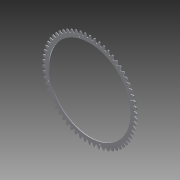
# Autodesk Inventor part: Large Spur Gear
Saved by Autodesk Inventor 2014 SP1 (Build 180222100, 222)
## iProperties
Created: 2012-03-30
Part Number: Large Spur Gear
Material: Aluminum-6061
Document SubType Name: Modeling
Designer: Moses
Mass: 183.263 g
Surface Area: 529.591 cm^2
Volume: 67.6246 cm^3
Density: 2.71 g/cm^3
Appearance: Aluminum - Flat
Author: Moses
Autodesk Inventor part; units mm, degrees
ref_plane "YZ Plane" through (0, 0, 0) normal (1, 0, 0) x (0, 1, 0)
ref_plane "XZ Plane" through (0, 0, 0) normal (0, 1, 0) x (-1, 0, 0)
ref_plane "XY Plane" through (0, 0, 0) normal (0, 0, 1) x (1, 0, 0)
sketch "Sketch1" plane through (0, 0, 0) normal (0, 0, 1) x (1, 0, 0)
  arc A0 (-21.3828, 186.7398) -> (-24.453, 174.3486) centre (39.2428, 165.1423) ccw
  arc A1 (-24.453, 174.3486) -> (-28.8619, 173.6732) centre (0, 0) ccw
  arc A2 (-28.8619, 173.6732) -> (-35.5008, 184.577) centre (-86.8806, 145.8209) ccw
  arc A3 (-35.5008, 184.577) -> (-40.1653, 183.6184) centre (0, 0) ccw
  arc A4 (-40.1653, 183.6184) -> (-41.9661, 170.9802) centre (22.3343, 168.2651) ccw
  arc A5 (-41.9661, 170.9802) -> (-46.2841, 169.8622) centre (0, 0) ccw
  arc A6 (-46.2841, 169.8622) -> (-53.992, 180.0384) centre (-101.1873, 136.2831) ccw
  arc A7 (-53.992, 180.0384) -> (-58.5355, 178.6129) centre (0, 0) ccw
  arc A8 (-58.5355, 178.6129) -> (-59.0486, 165.8573) centre (5.1966, 169.6613) ccw
  arc A9 (-59.0486, 165.8573) -> (-63.2313, 164.3082) centre (0, 0) ccw
  arc A10 (-63.2313, 164.3082) -> (-71.9292, 173.6524) centre (-114.4557, 125.347) ccw
  arc A11 (-71.9292, 173.6524) -> (-76.3052, 171.7745) centre (0, 0) ccw
  arc A12 (-76.3052, 171.7745) -> (-75.5251, 159.0325) centre (-11.9944, 169.3166) ccw
  arc A13 (-75.5251, 159.0325) -> (-79.5296, 157.0682) centre (0, 0) ccw
  arc A14 (-79.5296, 157.0682) -> (-89.1283, 165.4845) centre (-126.5496, 113.1245) ccw
  arc A15 (-89.1283, 165.4845) -> (-93.2918, 163.1735) centre (0, 0) ccw
  arc A16 (-93.2918, 163.1735) -> (-91.2267, 150.5758) centre (-29.0623, 167.2344) ccw
  arc A17 (-91.2267, 150.5758) -> (-95.0119, 148.2164) centre (0, 0) ccw
  arc A18 (-95.0119, 148.2164) -> (-105.4128, 155.6185) centre (-137.3449, 99.7413) ccw
  arc A19 (-105.4128, 155.6185) -> (-109.3212, 152.8982) centre (0, 0) ccw
  arc A20 (-109.3212, 152.8982) -> (-105.9921, 140.574) centre (-45.832, 163.4362) ccw
  arc A21 (-105.9921, 140.574) -> (-109.5192, 137.8438) centre (0, 0) ccw
  arc A22 (-109.5192, 137.8438) -> (-120.6156, 144.1556) centre (-146.7309, 85.3346) ccw
  arc A23 (-120.6156, 144.1556) -> (-124.2287, 141.0538) centre (0, 0) ccw
  arc A24 (-124.2287, 141.0538) -> (-119.67, 129.1297) centre (-62.1314, 157.9609) ccw
  arc A25 (-119.67, 129.1297) -> (-122.9028, 126.0567) centre (0, 0) ccw
  arc A26 (-122.9028, 126.0567) -> (-134.5807, 131.2135) centre (-154.6113, 70.0523) ccw
  arc A27 (-134.5807, 131.2135) -> (-137.8615, 127.7621) centre (0, 0) ccw
  arc A28 (-137.8615, 127.7621) -> (-132.1198, 116.3604) centre (-77.7933, 150.8647) ccw
  arc A29 (-132.1198, 116.3604) -> (-135.0251, 112.9761) centre (0, 0) ccw
  arc A30 (-135.0251, 112.9761) -> (-147.1649, 116.925) centre (-160.9051, 54.0511) ccw
  arc A31 (-147.1649, 116.925) -> (-150.0797, 113.1594) centre (0, 0) ccw
  arc A32 (-150.0797, 113.1594) -> (-143.2139, 102.397) centre (-92.6569, 142.2205) ccw
  arc A33 (-143.2139, 102.397) -> (-145.762, 98.7361) centre (0, 0) ccw
  arc A34 (-145.762, 98.7361) -> (-158.2389, 101.4367) centre (-165.5478, 37.4953) ccw
  arc A35 (-158.2389, 101.4367) -> (-160.7578, 97.3955) centre (0, 0) ccw
  arc A36 (-160.7578, 97.3955) -> (-152.8385, 87.3829) centre (-106.5697, 132.1168) ccw
  arc A37 (-152.8385, 87.3829) -> (-155.0031, 83.4831) centre (0, 0) ccw
  arc A38 (-155.0031, 83.4831) -> (-167.6892, 84.9075) centre (-168.4917, 20.5547) ccw
  arc A39 (-167.6892, 84.9075) -> (-169.7864, 80.6322) centre (0, 0) ccw
  arc A40 (-169.7864, 80.6322) -> (-160.8947, 71.4722) centre (-119.389, 120.6575) ccw
  arc A41 (-160.8947, 71.4722) -> (-162.6536, 67.3733) centre (0, 0) ccw
  arc A42 (-162.6536, 67.3733) -> (-175.4188, 67.507) centre (-169.7068, 3.4032) ccw
  arc A43 (-175.4188, 67.507) -> (-177.0727, 63.0415) centre (0, 0) ccw
  arc A44 (-177.0727, 63.0415) -> (-167.2999, 54.828) centre (-130.9832, 107.9601) ccw
  arc A45 (-167.2999, 54.828) -> (-168.6352, 50.5723) centre (0, 0) ccw
  arc A46 (-168.6352, 50.5723) -> (-181.3484, 49.4138) centre (-169.1803, -13.7832) ccw
  arc A47 (-181.3484, 49.4138) -> (-182.542, 44.8039) centre (0, 0) ccw
  arc A48 (-182.542, 44.8039) -> (-171.9884, 37.6213) centre (-141.2333, 94.1548) ccw
  arc A49 (-171.9884, 37.6213) -> (-172.8863, 33.2523) centre (0, 0) ccw
  arc A50 (-172.8863, 33.2523) -> (-185.4171, 30.8136) centre (-166.9179, -30.8281) ccw
  arc A51 (-185.4171, 30.8136) -> (-186.1381, 26.1066) centre (0, 0) ccw
  arc A52 (-186.1381, 26.1066) -> (-174.9121, 20.0285) centre (-150.0341, 79.3834) ccw
  arc A53 (-174.9121, 20.0285) -> (-175.3633, 15.5911) centre (0, 0) ccw
  arc A54 (-175.3633, 15.5911) -> (-187.5831, 11.8972) centre (-162.9427, -47.5568) ccw
  arc A55 (-187.5831, 11.8972) -> (-187.8243, 7.1414) centre (0, 0) ccw
  arc A56 (-187.8243, 7.1414) -> (-176.0409, 2.2302) centre (-157.2954, 63.7974) ccw
  arc A57 (-176.0409, 2.2302) -> (-176.0409, -2.2302) centre (0, 0) ccw
  arc A58 (-176.0409, -2.2302) -> (-187.8243, -7.1414) centre (-157.2954, -63.7974) ccw
  arc A59 (-187.8243, -7.1414) -> (-187.5831, -11.8972) centre (0, 0) ccw
  arc A60 (-187.5831, -11.8972) -> (-175.3633, -15.5911) centre (-162.9427, 47.5568) ccw
  arc A61 (-175.3633, -15.5911) -> (-174.9121, -20.0285) centre (0, 0) ccw
  arc A62 (-174.9121, -20.0285) -> (-186.1381, -26.1066) centre (-150.0341, -79.3834) ccw
  arc A63 (-186.1381, -26.1066) -> (-185.4171, -30.8136) centre (0, 0) ccw
  arc A64 (-185.4171, -30.8136) -> (-172.8863, -33.2523) centre (-166.9179, 30.8281) ccw
  arc A65 (-172.8863, -33.2523) -> (-171.9884, -37.6213) centre (0, 0) ccw
  arc A66 (-171.9884, -37.6213) -> (-182.542, -44.8039) centre (-141.2333, -94.1548) ccw
  arc A67 (-182.542, -44.8039) -> (-181.3484, -49.4138) centre (0, 0) ccw
  arc A68 (-181.3484, -49.4138) -> (-168.6352, -50.5723) centre (-169.1803, 13.7832) ccw
  arc A69 (-168.6352, -50.5723) -> (-167.2999, -54.828) centre (0, 0) ccw
  arc A70 (-167.2999, -54.828) -> (-177.0727, -63.0415) centre (-130.9832, -107.9601) ccw
  arc A71 (-177.0727, -63.0415) -> (-175.4188, -67.507) centre (0, 0) ccw
  arc A72 (-175.4188, -67.507) -> (-162.6536, -67.3733) centre (-169.7068, -3.4032) ccw
  arc A73 (-162.6536, -67.3733) -> (-160.8947, -71.4722) centre (0, 0) ccw
  arc A74 (-160.8947, -71.4722) -> (-169.7864, -80.6322) centre (-119.389, -120.6575) ccw
  arc A75 (-169.7864, -80.6322) -> (-167.6892, -84.9075) centre (0, 0) ccw
  arc A76 (-167.6892, -84.9075) -> (-155.0031, -83.4831) centre (-168.4917, -20.5547) ccw
  arc A77 (-155.0031, -83.4831) -> (-152.8385, -87.3829) centre (0, 0) ccw
  arc A78 (-152.8385, -87.3829) -> (-160.7578, -97.3955) centre (-106.5697, -132.1168) ccw
  arc A79 (-160.7578, -97.3955) -> (-158.2389, -101.4367) centre (0, 0) ccw
  arc A80 (-158.2389, -101.4367) -> (-145.762, -98.7361) centre (-165.5478, -37.4953) ccw
  arc A81 (-145.762, -98.7361) -> (-143.2139, -102.397) centre (0, 0) ccw
  arc A82 (-143.2139, -102.397) -> (-150.0797, -113.1594) centre (-92.6569, -142.2205) ccw
  arc A83 (-150.0797, -113.1594) -> (-147.1649, -116.925) centre (0, 0) ccw
  arc A84 (-147.1649, -116.925) -> (-135.0251, -112.9761) centre (-160.9051, -54.0511) ccw
  arc A85 (-135.0251, -112.9761) -> (-132.1198, -116.3604) centre (0, 0) ccw
  arc A86 (-132.1198, -116.3604) -> (-137.8615, -127.7621) centre (-77.7933, -150.8647) ccw
  arc A87 (-137.8615, -127.7621) -> (-134.5807, -131.2135) centre (0, 0) ccw
  arc A88 (-134.5807, -131.2135) -> (-122.9028, -126.0567) centre (-154.6113, -70.0523) ccw
  arc A89 (-122.9028, -126.0567) -> (-119.67, -129.1297) centre (0, 0) ccw
  arc A90 (-119.67, -129.1297) -> (-124.2287, -141.0538) centre (-62.1314, -157.9609) ccw
  arc A91 (-124.2287, -141.0538) -> (-120.6156, -144.1556) centre (0, 0) ccw
  arc A92 (-120.6156, -144.1556) -> (-109.5192, -137.8438) centre (-146.7309, -85.3346) ccw
  arc A93 (-109.5192, -137.8438) -> (-105.9921, -140.574) centre (0, 0) ccw
  arc A94 (-105.9921, -140.574) -> (-109.3212, -152.8982) centre (-45.832, -163.4362) ccw
  arc A95 (-109.3212, -152.8982) -> (-105.4128, -155.6185) centre (0, 0) ccw
  arc A96 (-105.4128, -155.6185) -> (-95.0119, -148.2164) centre (-137.3449, -99.7413) ccw
  arc A97 (-95.0119, -148.2164) -> (-91.2267, -150.5758) centre (0, 0) ccw
  arc A98 (-91.2267, -150.5758) -> (-93.2918, -163.1735) centre (-29.0623, -167.2344) ccw
  arc A99 (-93.2918, -163.1735) -> (-89.1283, -165.4845) centre (0, 0) ccw
  arc A100 (-89.1283, -165.4845) -> (-79.5296, -157.0682) centre (-126.5496, -113.1245) ccw
  arc A101 (-79.5296, -157.0682) -> (-75.5251, -159.0325) centre (0, 0) ccw
  arc A102 (-75.5251, -159.0325) -> (-76.3052, -171.7745) centre (-11.9944, -169.3166) ccw
  arc A103 (-76.3052, -171.7745) -> (-71.9292, -173.6524) centre (0, 0) ccw
  arc A104 (-71.9292, -173.6524) -> (-63.2313, -164.3082) centre (-114.4557, -125.347) ccw
  arc A105 (-63.2313, -164.3082) -> (-59.0486, -165.8573) centre (0, 0) ccw
  arc A106 (-59.0486, -165.8573) -> (-58.5355, -178.6129) centre (5.1966, -169.6613) ccw
  arc A107 (-58.5355, -178.6129) -> (-53.992, -180.0384) centre (0, 0) ccw
  arc A108 (-53.992, -180.0384) -> (-46.2841, -169.8622) centre (-101.1873, -136.2831) ccw
  arc A109 (-46.2841, -169.8622) -> (-41.9661, -170.9802) centre (0, 0) ccw
  arc A110 (-41.9661, -170.9802) -> (-40.1653, -183.6184) centre (22.3343, -168.2651) ccw
  arc A111 (-40.1653, -183.6184) -> (-35.5008, -184.577) centre (0, 0) ccw
  arc A112 (-35.5008, -184.577) -> (-28.8619, -173.6732) centre (-86.8806, -145.8209) ccw
  arc A113 (-28.8619, -173.6732) -> (-24.453, -174.3486) centre (0, 0) ccw
  arc A114 (-24.453, -174.3486) -> (-21.3828, -186.7398) centre (39.2428, -165.1423) ccw
  arc A115 (-21.3828, -186.7398) -> (-16.6453, -187.2215) centre (0, 0) ccw
  arc A116 (-16.6453, -187.2215) -> (-11.1436, -175.702) centre (-71.6824, -153.8623) ccw
  arc A117 (-11.1436, -175.702) -> (-6.689, -175.9279) centre (0, 0) ccw
  arc A118 (-6.689, -175.9279) -> (-2.381, -187.9449) centre (55.7487, -160.3248) ccw
  arc A119 (-2.381, -187.9449) -> (2.381, -187.9449) centre (0, 0) ccw
  arc A120 (2.381, -187.9449) -> (6.689, -175.9279) centre (-55.7487, -160.3248) ccw
  arc A121 (6.689, -175.9279) -> (11.1436, -175.702) centre (0, 0) ccw
  arc A122 (11.1436, -175.702) -> (16.6453, -187.2215) centre (71.6824, -153.8623) ccw
  arc A123 (16.6453, -187.2215) -> (21.3828, -186.7398) centre (0, 0) ccw
  arc A124 (21.3828, -186.7398) -> (24.453, -174.3486) centre (-39.2428, -165.1423) ccw
  arc A125 (24.453, -174.3486) -> (28.8619, -173.6732) centre (0, 0) ccw
  arc A126 (28.8619, -173.6732) -> (35.5008, -184.577) centre (86.8806, -145.8209) ccw
  arc A127 (35.5008, -184.577) -> (40.1653, -183.6184) centre (0, 0) ccw
  arc A128 (40.1653, -183.6184) -> (41.9661, -170.9802) centre (-22.3343, -168.2651) ccw
  arc A129 (41.9661, -170.9802) -> (46.2841, -169.8622) centre (0, 0) ccw
  arc A130 (46.2841, -169.8622) -> (53.992, -180.0384) centre (101.1873, -136.2831) ccw
  arc A131 (53.992, -180.0384) -> (58.5355, -178.6129) centre (0, 0) ccw
  arc A132 (58.5355, -178.6129) -> (59.0486, -165.8573) centre (-5.1966, -169.6613) ccw
  arc A133 (59.0486, -165.8573) -> (63.2313, -164.3082) centre (0, 0) ccw
  arc A134 (63.2313, -164.3082) -> (71.9292, -173.6524) centre (114.4557, -125.347) ccw
  arc A135 (71.9292, -173.6524) -> (76.3052, -171.7745) centre (0, 0) ccw
  arc A136 (76.3052, -171.7745) -> (75.5251, -159.0325) centre (11.9944, -169.3166) ccw
  arc A137 (75.5251, -159.0325) -> (79.5296, -157.0682) centre (0, 0) ccw
  arc A138 (79.5296, -157.0682) -> (89.1283, -165.4845) centre (126.5496, -113.1245) ccw
  arc A139 (89.1283, -165.4845) -> (93.2918, -163.1735) centre (0, 0) ccw
  arc A140 (93.2918, -163.1735) -> (91.2267, -150.5758) centre (29.0623, -167.2344) ccw
  arc A141 (91.2267, -150.5758) -> (95.0119, -148.2164) centre (0, 0) ccw
  arc A142 (95.0119, -148.2164) -> (105.4128, -155.6185) centre (137.3449, -99.7413) ccw
  arc A143 (105.4128, -155.6185) -> (109.3212, -152.8982) centre (0, 0) ccw
  arc A144 (109.3212, -152.8982) -> (105.9921, -140.574) centre (45.832, -163.4362) ccw
  arc A145 (105.9921, -140.574) -> (109.5192, -137.8438) centre (0, 0) ccw
  arc A146 (109.5192, -137.8438) -> (120.6156, -144.1556) centre (146.7309, -85.3346) ccw
  arc A147 (120.6156, -144.1556) -> (124.2287, -141.0538) centre (0, 0) ccw
  arc A148 (124.2287, -141.0538) -> (119.67, -129.1297) centre (62.1314, -157.9609) ccw
  arc A149 (119.67, -129.1297) -> (122.9028, -126.0567) centre (0, 0) ccw
  arc A150 (122.9028, -126.0567) -> (134.5807, -131.2135) centre (154.6113, -70.0523) ccw
  arc A151 (134.5807, -131.2135) -> (137.8615, -127.7621) centre (0, 0) ccw
  arc A152 (137.8615, -127.7621) -> (132.1198, -116.3604) centre (77.7933, -150.8647) ccw
  arc A153 (132.1198, -116.3604) -> (135.0251, -112.9761) centre (0, 0) ccw
  arc A154 (135.0251, -112.9761) -> (147.1649, -116.925) centre (160.9051, -54.0511) ccw
  arc A155 (147.1649, -116.925) -> (150.0797, -113.1594) centre (0, 0) ccw
  arc A156 (150.0797, -113.1594) -> (143.2139, -102.397) centre (92.6569, -142.2205) ccw
  arc A157 (143.2139, -102.397) -> (145.762, -98.7361) centre (0, 0) ccw
  arc A158 (145.762, -98.7361) -> (158.2389, -101.4367) centre (165.5478, -37.4953) ccw
  arc A159 (158.2389, -101.4367) -> (160.7578, -97.3955) centre (0, 0) ccw
  arc A160 (160.7578, -97.3955) -> (152.8385, -87.3829) centre (106.5697, -132.1168) ccw
  arc A161 (152.8385, -87.3829) -> (155.0031, -83.4831) centre (0, 0) ccw
  arc A162 (155.0031, -83.4831) -> (167.6892, -84.9075) centre (168.4917, -20.5547) ccw
  arc A163 (167.6892, -84.9075) -> (169.7864, -80.6322) centre (0, 0) ccw
  arc A164 (169.7864, -80.6322) -> (160.8947, -71.4722) centre (119.389, -120.6575) ccw
  arc A165 (160.8947, -71.4722) -> (162.6536, -67.3733) centre (0, 0) ccw
  arc A166 (162.6536, -67.3733) -> (175.4188, -67.507) centre (169.7068, -3.4032) ccw
  arc A167 (175.4188, -67.507) -> (177.0727, -63.0415) centre (0, 0) ccw
  arc A168 (177.0727, -63.0415) -> (167.2999, -54.828) centre (130.9832, -107.9601) ccw
  arc A169 (167.2999, -54.828) -> (168.6352, -50.5723) centre (0, 0) ccw
  arc A170 (168.6352, -50.5723) -> (181.3484, -49.4138) centre (169.1803, 13.7832) ccw
  arc A171 (181.3484, -49.4138) -> (182.542, -44.8039) centre (0, 0) ccw
  arc A172 (182.542, -44.8039) -> (171.9884, -37.6213) centre (141.2333, -94.1548) ccw
  arc A173 (171.9884, -37.6213) -> (172.8863, -33.2523) centre (0, 0) ccw
  arc A174 (172.8863, -33.2523) -> (185.4171, -30.8136) centre (166.9179, 30.8281) ccw
  arc A175 (185.4171, -30.8136) -> (186.1381, -26.1066) centre (0, 0) ccw
  arc A176 (186.1381, -26.1066) -> (174.9121, -20.0285) centre (150.0341, -79.3834) ccw
  arc A177 (174.9121, -20.0285) -> (175.3633, -15.5911) centre (0, 0) ccw
  arc A178 (175.3633, -15.5911) -> (187.5831, -11.8972) centre (162.9427, 47.5568) ccw
  arc A179 (187.5831, -11.8972) -> (187.8243, -7.1414) centre (0, 0) ccw
  arc A180 (187.8243, -7.1414) -> (176.0409, -2.2302) centre (157.2954, -63.7974) ccw
  arc A181 (176.0409, -2.2302) -> (176.0409, 2.2302) centre (0, 0) ccw
  arc A182 (176.0409, 2.2302) -> (187.8243, 7.1414) centre (157.2954, 63.7974) ccw
  arc A183 (187.8243, 7.1414) -> (187.5831, 11.8972) centre (0, 0) ccw
  arc A184 (187.5831, 11.8972) -> (175.3633, 15.5911) centre (162.9427, -47.5568) ccw
  arc A185 (175.3633, 15.5911) -> (174.9121, 20.0285) centre (0, 0) ccw
  arc A186 (174.9121, 20.0285) -> (186.1381, 26.1066) centre (150.0341, 79.3834) ccw
  arc A187 (186.1381, 26.1066) -> (185.4171, 30.8136) centre (0, 0) ccw
  arc A188 (185.4171, 30.8136) -> (172.8863, 33.2523) centre (166.9179, -30.8281) ccw
  arc A189 (172.8863, 33.2523) -> (171.9884, 37.6213) centre (0, 0) ccw
  arc A190 (171.9884, 37.6213) -> (182.542, 44.8039) centre (141.2333, 94.1548) ccw
  arc A191 (182.542, 44.8039) -> (181.3484, 49.4138) centre (0, 0) ccw
  arc A192 (181.3484, 49.4138) -> (168.6352, 50.5723) centre (169.1803, -13.7832) ccw
  arc A193 (168.6352, 50.5723) -> (167.2999, 54.828) centre (0, 0) ccw
  arc A194 (167.2999, 54.828) -> (177.0727, 63.0415) centre (130.9832, 107.9601) ccw
  arc A195 (177.0727, 63.0415) -> (175.4188, 67.507) centre (0, 0) ccw
  arc A196 (175.4188, 67.507) -> (162.6536, 67.3733) centre (169.7068, 3.4032) ccw
  arc A197 (162.6536, 67.3733) -> (160.8947, 71.4722) centre (0, 0) ccw
  arc A198 (160.8947, 71.4722) -> (169.7864, 80.6322) centre (119.389, 120.6575) ccw
  arc A199 (169.7864, 80.6322) -> (167.6892, 84.9075) centre (0, 0) ccw
  arc A200 (167.6892, 84.9075) -> (155.0031, 83.4831) centre (168.4917, 20.5547) ccw
  arc A201 (155.0031, 83.4831) -> (152.8385, 87.3829) centre (0, 0) ccw
  arc A202 (152.8385, 87.3829) -> (160.7578, 97.3955) centre (106.5697, 132.1168) ccw
  arc A203 (160.7578, 97.3955) -> (158.2389, 101.4367) centre (0, 0) ccw
  arc A204 (158.2389, 101.4367) -> (145.762, 98.7361) centre (165.5478, 37.4953) ccw
  arc A205 (145.762, 98.7361) -> (143.2139, 102.397) centre (0, 0) ccw
  arc A206 (143.2139, 102.397) -> (150.0797, 113.1594) centre (92.6569, 142.2205) ccw
  arc A207 (150.0797, 113.1594) -> (147.1649, 116.925) centre (0, 0) ccw
  arc A208 (147.1649, 116.925) -> (135.0251, 112.9761) centre (160.9051, 54.0511) ccw
  arc A209 (135.0251, 112.9761) -> (132.1198, 116.3604) centre (0, 0) ccw
  arc A210 (132.1198, 116.3604) -> (137.8615, 127.7621) centre (77.7933, 150.8647) ccw
  arc A211 (137.8615, 127.7621) -> (134.5807, 131.2135) centre (0, 0) ccw
  arc A212 (134.5807, 131.2135) -> (122.9028, 126.0567) centre (154.6113, 70.0523) ccw
  arc A213 (122.9028, 126.0567) -> (119.67, 129.1297) centre (0, 0) ccw
  arc A214 (119.67, 129.1297) -> (124.2287, 141.0538) centre (62.1314, 157.9609) ccw
  arc A215 (124.2287, 141.0538) -> (120.6156, 144.1556) centre (0, 0) ccw
  arc A216 (120.6156, 144.1556) -> (109.5192, 137.8438) centre (146.7309, 85.3346) ccw
  arc A217 (109.5192, 137.8438) -> (105.9921, 140.574) centre (0, 0) ccw
  arc A218 (105.9921, 140.574) -> (109.3212, 152.8982) centre (45.832, 163.4362) ccw
  arc A219 (109.3212, 152.8982) -> (105.4128, 155.6185) centre (0, 0) ccw
  arc A220 (105.4128, 155.6185) -> (95.0119, 148.2164) centre (137.3449, 99.7413) ccw
  arc A221 (95.0119, 148.2164) -> (91.2267, 150.5758) centre (0, 0) ccw
  arc A222 (91.2267, 150.5758) -> (93.2918, 163.1735) centre (29.0623, 167.2344) ccw
  arc A223 (93.2918, 163.1735) -> (89.1283, 165.4845) centre (0, 0) ccw
  arc A224 (89.1283, 165.4845) -> (79.5296, 157.0682) centre (126.5496, 113.1245) ccw
  arc A225 (79.5296, 157.0682) -> (75.5251, 159.0325) centre (0, 0) ccw
  arc A226 (75.5251, 159.0325) -> (76.3052, 171.7745) centre (11.9944, 169.3166) ccw
  arc A227 (76.3052, 171.7745) -> (71.9292, 173.6524) centre (0, 0) ccw
  arc A228 (71.9292, 173.6524) -> (63.2313, 164.3082) centre (114.4557, 125.347) ccw
  arc A229 (63.2313, 164.3082) -> (59.0486, 165.8573) centre (0, 0) ccw
  arc A230 (59.0486, 165.8573) -> (58.5355, 178.6129) centre (-5.1966, 169.6613) ccw
  arc A231 (58.5355, 178.6129) -> (53.992, 180.0384) centre (0, 0) ccw
  arc A232 (53.992, 180.0384) -> (46.2841, 169.8622) centre (101.1873, 136.2831) ccw
  arc A233 (46.2841, 169.8622) -> (41.9661, 170.9802) centre (0, 0) ccw
  arc A234 (41.9661, 170.9802) -> (40.1653, 183.6184) centre (-22.3343, 168.2651) ccw
  arc A235 (40.1653, 183.6184) -> (35.5008, 184.577) centre (0, 0) ccw
  arc A236 (35.5008, 184.577) -> (28.8619, 173.6732) centre (86.8806, 145.8209) ccw
  arc A237 (28.8619, 173.6732) -> (24.453, 174.3486) centre (0, 0) ccw
  arc A238 (24.453, 174.3486) -> (21.3828, 186.7398) centre (-39.2428, 165.1423) ccw
  arc A239 (21.3828, 186.7398) -> (16.6453, 187.2215) centre (0, 0) ccw
  arc A240 (16.6453, 187.2215) -> (11.1436, 175.702) centre (71.6824, 153.8623) ccw
  arc A241 (11.1436, 175.702) -> (6.689, 175.9279) centre (0, 0) ccw
  arc A242 (6.689, 175.9279) -> (2.381, 187.9449) centre (-55.7487, 160.3248) ccw
  arc A243 (2.381, 187.9449) -> (-2.381, 187.9449) centre (0, 0) ccw
  arc A244 (-2.381, 187.9449) -> (-6.689, 175.9279) centre (55.7487, 160.3248) ccw
  arc A245 (-6.689, 175.9279) -> (-11.1436, 175.702) centre (0, 0) ccw
  arc A246 (-11.1436, 175.702) -> (-16.6453, 187.2215) centre (-71.6824, 153.8623) ccw
  arc A247 (-16.6453, 187.2215) -> (-21.3828, 186.7398) centre (0, 0) ccw
  point P0 (0, 0)
  constraints: 496 point on circle, 248 centre point, 745 other
extrude "Extrusion1" add sketch "Sketch1" along normal blind 3.175
sketch "Sketch2" plane through (0, 0, 3.175) normal (0, 0, 1) x (1, 0, 0)
  circle A0 centre (0, 0) radius 162.5 projected
extrude "Extrusion2" cut sketch "Sketch2" against normal blind 25.4
sketch "Sketch3" plane through (0, 0, 0) normal (0, 0, -1) x (-1, 0, 0)
  circle A0 centre (39.8868, 165.864) radius 3.3782 projected
  circle A1 centre (-163.5858, 48.389) radius 3.3782 projected
  circle A2 centre (-39.8868, -165.864) radius 3.3782 projected
  circle A3 centre (163.5858, -48.389) radius 3.3782 projected
extrude "Extrusion3" cut sketch "Sketch3" against normal blind 25.4
equation "\"BendRadius\" = Thickness"
equation "\"BendReliefWidth\" = Thickness"
equation "\"BendReliefDepth\" = 0.5 * Thickness"
equation "\"CornerReliefSize\" = 4 * Thickness"
equation "\"MinimumRemnant\" = 2 * Thickness"
equation "\"TransitionRadius\" = BendRadius"
equation "\"JacobiRadiusSize\" = Thickness"
equation "\"GapSize\" = Thickness"
equation "\"Thickness\" = 3.048"
body "Solid1"
